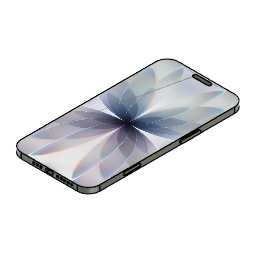
iPhone_17 (Autodesk Fusion 360 design; units mm, degrees)
Autodesk Fusion 360 part; units mm, degrees
sketch "Sketch1" plane through (0, 0, 0) normal (0, 0, 1) x (1, 0, 0)
  line L0 (140, 280) -> (-140, 280)
  line L1 (-140, 280) -> (-140, -280)
  line L2 (-140, -280) -> (140, -280)
  line L3 (140, -280) -> (140, 280)
  line L4 (140, 280) -> (-140, -280) construction
  line L5 (-140, 280) -> (140, -280) construction
  dimension "d1" = 140
  dimension "d2" = 280
  constraint horizontal L0
  constraint perpendicular L0 L1
  constraint parallel L0 L2
  constraint parallel L1 L3
  constraint coincident L4 origin
  constraint coincident L5 origin
  measures "d1" distance of origin L1
  measures "d2" distance of origin L2
extrude "Extrude1" add sketch "Sketch1" along normal blind 20
fillet "Fillet1" radius 40 4 edges at (140, -280, 10) (-140, -280, 10) (140, 280, 10) (-140, 280, 10)
sketch "Sketch2" plane through (0, -280, 0) normal (0, -1, 0) x (1, 0, 0)
  line L0 (-100, 20) -> (-100, 0)
  line L1 (-100, 0) -> (100, 0)
  line L2 (100, 0) -> (100, 20)
  line L3 (100, 20) -> (-100, 20)
  line L4 (10, 15) -> (-10, 15)
  line L5 (-10, 5) -> (10, 5)
  line L6 (10, 15) -> (-10, 5) construction
  line L7 (-10, 15) -> (10, 5) construction
  arc A0 (10, 5) -> (10, 15) centre (8.875, 10) ccw
  line L8 (0, 15) -> (0, 5) construction
  arc A1 (-10, 15) -> (-10, 5) centre (-8.875, 10) ccw
  circle A2 centre (-30, 10) radius 3.8849
  circle A3 centre (-42.5, 10) radius 3.8849
  circle A4 centre (-55, 10) radius 3.8849
  circle A5 centre (30, 10) radius 3.8849
  circle A6 centre (42.5, 10) radius 3.8849
  circle A7 centre (55, 10) radius 3.8849
  circle A8 centre (67.5, 10) radius 3.8849
  circle A9 centre (80, 10) radius 3.8849
  point P0 (0, 10)
  dimension "d7" = 20
  dimension "d8" = 5.125
  dimension "d9" = 10
  dimension "d10" = 5
  dimension "d11" = 100
  dimension "d12" = 10
  dimension "d17" = -25
  dimension "d18" = 0
  dimension "d21" = 50
  dimension "d22" = 0
  constraint horizontal L4
  constraint parallel L4 L5
  constraint coincident L6 P0
  constraint coincident L7 P0
  constraint midpoint L4 L8.start
  constraint midpoint L5 L8.end
  constraint symmetric L4.start L8 L4.end
  constraint symmetric L5.end L8 L5.start
  constraint symmetric A0 L8 A1
  constraint coincident L5.start L6.end
  constraint symmetric L8 A2 A5
  measures "d7" distance of L5.end L5.start
  measures "d8" radius of A0
  measures "d9" distance of L1 A0.centre
  measures "d10" distance of L5 A0.centre
  measures "d11" distance of L0.end L8
  measures "d12" distance of L4 L5
extrude "Extrude2" cut sketch "Sketch2" against normal blind 13 contours L4 L5 A0 A1
extrude "Extrude3" cut sketch "Sketch2" against normal blind 2 contours A2 | A3 | A4 | A5 | A6 | A7 | A8 | A9
sketch "Sketch3" plane through (140, 0, 0) normal (1, 0, 0) x (0, 1, 0)
  line L0 (240, 0) -> (240, 20)
  line L1 (240, 20) -> (-240, 20)
  line L2 (-240, 20) -> (-240, 0)
  line L3 (-240, 0) -> (240, 0)
  line L4 (-150, 4.2611) -> (-100, 4.2611)
  arc A0 (-100, 4.2611) -> (-100, 15.7389) centre (-100, 10) ccw
  line L5 (-100, 15.7389) -> (-150, 15.7389)
  arc A1 (-150, 15.7389) -> (-150, 4.2611) centre (-150, 10) ccw
  line L6 (-150, 10) -> (-100, 10) construction
  line L7 (50, 4.2841) -> (110, 4.2841)
  arc A2 (110, 4.2841) -> (110, 15.7159) centre (110, 10) ccw
  line L8 (110, 15.7159) -> (50, 15.7159)
  arc A3 (50, 15.7159) -> (50, 4.2841) centre (50, 10) ccw
  line L9 (50, 10) -> (110, 10) construction
  dimension "d27" = 11.4319
  constraint tangent L4 A0
  constraint tangent A0 L5
  constraint parallel L4 L5
  constraint tangent L5 A1
  constraint tangent L4 A1
  constraint parallel L1 L6
  constraint tangent L7 A2
  constraint tangent A2 L8
  constraint parallel L7 L8
  constraint tangent L8 A3
  constraint tangent L7 A3
  constraint parallel L1 L9
  measures "d27" distance of L7.end A2.end
extrude "Extrude4" cut sketch "Sketch3" against normal blind 1 contours L4 A0 L5 A1
extrude "Extrude5" add sketch "Sketch3" along normal blind 5 contours L7 A2 L8 A3
sketch "Sketch4" plane through (-140, 0, 0) normal (-1, 0, 0) x (0, -1, 0)
  line L0 (-240, 20) -> (-240, 0)
  line L1 (-240, 0) -> (240, 0)
  line L2 (240, 0) -> (240, 20)
  line L3 (240, 20) -> (-240, 20)
  line L4 (-130, 4.0036) -> (-90, 4.0036)
  arc A0 (-90, 4.0036) -> (-90, 15.9964) centre (-90, 10) ccw
  line L5 (-90, 15.9964) -> (-130, 15.9964)
  arc A1 (-130, 15.9964) -> (-130, 4.0036) centre (-130, 10) ccw
  line L6 (-130, 10) -> (-90, 10) construction
  line L7 (-77.5677, 20) -> (-77.5677, 0) construction
  arc A2 (-65.1354, 15.9964) -> (-65.1354, 4.0036) centre (-65.1354, 10) ccw
  line L8 (-65.1354, 15.9964) -> (-25.1354, 15.9964)
  arc A3 (-25.1354, 4.0036) -> (-25.1354, 15.9964) centre (-25.1354, 10) ccw
  line L9 (-25.1354, 4.0036) -> (-65.1354, 4.0036)
  line L10 (-177, 4.5) -> (-170, 4.5)
  arc A4 (-170, 4.5) -> (-170, 15.5) centre (-170, 10) ccw
  line L11 (-170, 15.5) -> (-177, 15.5)
  arc A5 (-177, 15.5) -> (-177, 4.5) centre (-177, 10) ccw
  line L12 (-177, 10) -> (-170, 10) construction
  dimension "d30" = 40
  dimension "d31" = 11
  constraint tangent L4 A0
  constraint tangent A0 L5
  constraint parallel L4 L5
  constraint tangent L5 A1
  constraint tangent L4 A1
  constraint parallel L3 L6
  constraint coincident L3 L7.start
  constraint coincident L1 L7.end
  constraint perpendicular L1 L7
  constraint symmetric L4.start L7 A3.start
  constraint symmetric L4.end L7 A2.end
  constraint symmetric A0.end L7 A2.start
  constraint symmetric L5.end L7 L8.end
  constraint symmetric A0 L7 A2
  constraint symmetric A1 L7 A3
  constraint tangent L10 A4
  constraint tangent A4 L11
  constraint parallel L10 L11
  constraint tangent L11 A5
  constraint tangent L10 A5
  constraint parallel L6 L12
  measures "d30" distance of A1.centre A0.centre
  measures "d31" diameter of A4
extrude "Extrude6" add sketch "Sketch4" along normal blind 4 contours L4 A0 L5 A1 | A2 L8 A3 L9 | L10 A4 L11 A5
sketch "Sketch5" plane through (0, 0, 0) normal (0, 0, -1) x (1, 0, 0)
  arc A0 (-140, -240) -> (-100, -280) centre (-100, -240) ccw
  line L0 (-100, -280) -> (100, -280)
  arc A1 (100, -280) -> (140, -240) centre (100, -240) ccw
  line L1 (140, -240) -> (140, 240)
  arc A2 (140, 240) -> (100, 280) centre (100, 240) ccw
  line L2 (100, 280) -> (-100, 280)
  arc A3 (-100, 280) -> (-140, 240) centre (-100, 240) ccw
  line L3 (-140, 240) -> (-140, -240)
  line L4 (126.7816, -230) -> (126.7816, -165)
  arc A4 (126.7816, -165) -> (56.6683, -165) centre (91.725, -165) ccw
  line L5 (56.6683, -165) -> (56.6683, -230)
  arc A5 (56.6683, -230) -> (126.7816, -230) centre (91.725, -230) ccw
  line L6 (91.725, -230) -> (91.725, -165) construction
  dimension "d34" = 35.0567
  dimension "d36" = 75
  dimension "d38" = 50
  constraint tangent L4 A4
  constraint tangent A4 L5
  constraint parallel L4 L5
  constraint tangent L5 A5
  constraint tangent L4 A5
  constraint vertical L6
  measures "d34" radius of A5
  measures "d36" vertical distance of A0.centre A4.centre
  measures "d38" distance of L0 A5.centre
extrude "Extrude7" add sketch "Sketch5" along normal blind 5 contours L4 A4 L5 A5
sketch "Sketch6" plane through (0, 0, -5) normal (0, 0, -1) x (1, 0, 0)
  arc A0 (56.6683, -230) -> (126.7816, -230) centre (91.725, -230) ccw
  line L0 (126.7816, -230) -> (126.7816, -165)
  arc A1 (126.7816, -165) -> (56.6683, -165) centre (91.725, -165) ccw
  line L1 (56.6683, -165) -> (56.6683, -230)
  circle A2 centre (91.725, -230) radius 28.5736
  line L2 (91.725, -197.5847) -> (60, -197.5847) construction
  circle A3 centre (91.725, -165.1693) radius 28.5736
  constraint concentric A0 A2
  constraint perpendicular L1 L2
  constraint symmetric A2 L2 A3
extrude "Extrude8" add sketch "Sketch6" along normal blind 5 contours A2 | A3
sketch "Sketch7" plane through (0, 0, 0) normal (0, 0, -1) x (1, 0, 0)
  line L0 (56.6683, -230) -> (56.6683, -165)
  arc A0 (126.7816, -165) -> (56.6683, -165) centre (91.725, -165) ccw
  line L1 (126.7816, -165) -> (126.7816, -230)
  arc A1 (56.6683, -230) -> (126.7816, -230) centre (91.725, -230) ccw
  arc A2 (-140, -240) -> (-100, -280) centre (-100, -240) ccw
  line L2 (-100, -280) -> (100, -280)
  arc A3 (100, -280) -> (140, -240) centre (100, -240) ccw
  line L3 (140, -240) -> (140, 240)
  arc A4 (140, 240) -> (100, 280) centre (100, 240) ccw
  line L4 (100, 280) -> (-100, 280)
  arc A5 (-100, 280) -> (-140, 240) centre (-100, 240) ccw
  line L5 (-140, 240) -> (-140, -240)
  circle A6 centre (35.4902, -197.5) radius 7.4639
extrude "Extrude9" add sketch "Sketch7" along normal blind 1.5 contours A6
sketch "Sketch8" plane through (0, 0, 20) normal (0, 0, 1) x (-1, 0, 0)
  arc A0 (100, -280) -> (140, -240) centre (100, -240) ccw
  line L0 (140, -240) -> (140, 240)
  arc A1 (140, 240) -> (100, 280) centre (100, 240) ccw
  line L1 (100, 280) -> (-100, 280)
  arc A2 (-100, 280) -> (-140, 240) centre (-100, 240) ccw
  line L2 (-140, 240) -> (-140, -240)
  arc A3 (-140, -240) -> (-100, -280) centre (-100, -240) ccw
  line L3 (-100, -280) -> (100, -280)
  line L4 (25, -258.4273) -> (-25, -258.4273)
  arc A4 (-25, -258.4273) -> (-25, -271.5727) centre (-25, -265) ccw
  line L5 (-25, -271.5727) -> (25, -271.5727)
  arc A5 (25, -271.5727) -> (25, -258.4273) centre (25, -265) ccw
  line L6 (25, -265) -> (-25, -265) construction
  constraint tangent L4 A4
  constraint tangent A4 L5
  constraint parallel L4 L5
  constraint tangent L5 A5
  constraint tangent L4 A5
  constraint horizontal L6
extrude "Extrude10" add sketch "Sketch8" along normal blind 1 contours L4 A4 L5 A5
sketch "Sketch9" plane through (0, 0, 0) normal (0, 0, -1) x (1, 0, 0)
  circle A0 centre (35.4902, -197.5) radius 7.4639
  line L0 (56.6683, -230) -> (56.6683, -165)
  arc A1 (126.7816, -165) -> (56.6683, -165) centre (91.725, -165) ccw
  line L1 (126.7816, -165) -> (126.7816, -230)
  arc A2 (56.6683, -230) -> (126.7816, -230) centre (91.725, -230) ccw
  arc A3 (-140, -240) -> (-100, -280) centre (-100, -240) ccw
  line L2 (-100, -280) -> (100, -280)
  arc A4 (100, -280) -> (140, -240) centre (100, -240) ccw
  line L3 (140, -240) -> (140, 240)
  arc A5 (140, 240) -> (100, 280) centre (100, 240) ccw
  line L4 (100, 280) -> (-100, 280)
  arc A6 (-100, 280) -> (-140, 240) centre (-100, 240) ccw
  line L5 (-140, 240) -> (-140, -240)
  spline S0 degree 3 poles (-24.7768, 20.7597) (-21.4828, 25.6809) (-17.9903, 30.4831) (-12.6722, 30.5625) knots 0 0 0 0 1 1 1 1
  spline S1 degree 3 poles (-12.6722, 30.5625) (-7.354, 30.6815) (-5.6475, 27.4272) (0.385, 27.4272) knots 0 0 0 0 1 1 1 1
  spline S2 degree 3 poles (0.385, 27.4272) (6.4572, 27.4272) (8.3225, 30.4831) (13.363, 30.6815) knots 0 0 0 0 1 1 1 1
  spline S3 degree 3 poles (13.363, 30.6815) (18.562, 30.88) (22.4911, 25.4428) (25.8248, 20.6406) knots 0 0 0 0 1 1 1 1
  spline S4 degree 3 poles (25.8248, 20.6406) (32.6114, 10.8378) (37.8105, -7.22) (30.8255, -19.3644) knots 0 0 0 0 1 1 1 1
  spline S5 degree 3 poles (30.8255, -19.3644) (27.3726, -25.3969) (21.1814, -29.2069) (14.4742, -29.326) knots 0 0 0 0 1 1 1 1
  spline S6 degree 3 poles (14.4742, -29.326) (9.3941, -29.4053) (4.5522, -25.8731) (1.4169, -25.8731) knots 0 0 0 0 1 1 1 1
  spline S7 degree 3 poles (1.4169, -25.8731) (-1.6787, -25.8731) (-7.5525, -30.1197) (-13.704, -29.4847) knots 0 0 0 0 1 1 1 1
  spline S8 degree 3 poles (-13.704, -29.4847) (-16.2837, -29.3657) (-23.5068, -28.4528) (-28.1503, -21.6266) knots 0 0 0 0 1 1 1 1
  spline S9 degree 3 poles (-28.1503, -21.6266) (-27.7931, -21.3885) (-19.5381, -16.5466) (-19.6175, -6.5056) knots 0 0 0 0 1 1 1 1
  spline S10 degree 3 poles (-19.6175, -6.5056) (-19.7365, 5.48) (-30.1347, 9.4884) (-30.2537, 9.5281) knots 0 0 0 0 1 1 1 1
  spline S11 degree 3 poles (-30.2537, 9.5281) (-30.1347, 9.8059) (-28.5868, 15.2431) (-24.7768, 20.7597) knots 0 0 0 0 1 1 1 1
  spline S12 degree 3 poles (-2.1153, -42.7403) (-5.0125, -46.0344) (-9.8147, -48.5347) (-13.7834, -48.6935) knots 0 0 0 0 1 1 1 1
  spline S13 degree 3 poles (-13.7834, -48.6935) (-14.2993, -44.05) (-12.434, -39.3669) (-9.6559, -36.0331) knots 0 0 0 0 1 1 1 1
  spline S14 degree 3 poles (-9.6559, -36.0331) (-6.9175, -32.6597) (-2.3931, -30.0403) (2.0519, -30.3975) knots 0 0 0 0 1 1 1 1
  spline S15 degree 3 poles (2.0519, -30.3975) (2.6472, -34.9616) (0.4247, -39.7241) (-2.1153, -42.7403) knots 0 0 0 0 1 1 1 1
